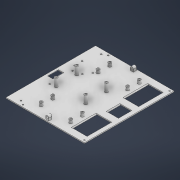
# Autodesk Inventor part: Obenplatte_hinten
Saved by Autodesk Inventor 2021 (Build 250183000, 183)
## iProperties
Created: 2021-02-01
Part Number: Obenplatte_hinten
Material: Generisch
Document SubType Name: Modeling
Designer: laure
Density: 1 g/cm^3
Appearance: Vorgabe
Author: laure
## iProperties of the stored document _3D-Druck.ipt
Created: 2021-02-04
Part Number: _3D-Druck
Material: Generisch
Document SubType Name: Modeling
Designer: Ctroi
Density: 1 g/cm^3
Appearance: Vorgabe
Author: Ctroi
Autodesk Inventor part; units mm, degrees
ref_plane "YZ Plane" through (0, 0, 0) normal (1, 0, 0) x (0, 1, 0)
ref_plane "XZ Plane" through (0, 0, 0) normal (0, 1, 0) x (-1, 0, 0)
ref_plane "XY Plane" through (0, 0, 0) normal (0, 0, 1) x (1, 0, 0)
sketch "Skizze1" plane through (0, 0, 0) normal (0, 1, 0) x (-1, 0, 0)
  line L0 (87.5, -100) -> (-87.5, -100)
  line L1 (-87.5, -100) -> (-87.5, 100)
  line L2 (-87.5, 100) -> (87.5, 100)
  line L3 (87.5, 100) -> (87.5, -100)
  line L4 (0, -140) -> (0, 140) projected
  line L5 (-122.5, 0) -> (122.5, 0) projected
  point P0 (0, 0)
  dimension "d0" = 175
  dimension "d1" = 200
  constraints: 8 end point, 2 parallel, 1 horizontal, 1 perpendicular, 2 other
  measures "d0" distance of L1.end L2.end
  measures "d1" distance of L0.end L1.end
extrude "Extrusion1" add sketch "Skizze1" along normal blind 2
sketch "Skizze2" plane through (0, 2, 0) normal (0, 1, 0) x (1, 0, 0)
  circle A0 centre (-54.5, 95) radius 1.6
  line L0 (0, 140) -> (0, -140) projected
  line L1 (122.5, 0) -> (-122.5, 0) projected
  line L2 (87.5, 100) -> (-87.5, 100) projected
  circle A1 centre (82.5, 95) radius 1.6
  circle A2 centre (-54.5, -95) radius 1.6
  circle A3 centre (82.5, -95) radius 1.6
  line L3 (-87.5, 100) -> (-87.5, -100) projected
  line L4 (87.5, -100) -> (87.5, 100) projected
  point P0 (0, 0)
  dimension "d4" = 3.2
  dimension "d6" = 5
  dimension "d7" = 3.2
  dimension "d9" = 5
  dimension "d40" = 33
  dimension "d41" = 5
  constraints: 4 centre point, 2 symmetric about line, 2 other
  measures "d4" diameter of A0
  measures "d6" distance from line of A0.centre L2
  measures "d7" diameter of A1
  measures "d9" distance from line of L2 A1.centre
  measures "d40" distance from line of L3 A0.centre
  measures "d41" distance from line of L4 A1.centre
extrude "Extrusion2" cut sketch "Skizze2" against normal up to surface (2 mm away) contours A0 | A1 | A2 | A3
sketch "Skizze3" plane through (0, 2, 0) normal (0, 1, 0) x (1, 0, 0)
  line L0 (87.5, -100) -> (87.5, 100) projected
  line L1 (-87.5, -100) -> (87.5, -100) projected
  line L2 (87.5, 100) -> (-87.5, 100) projected
  circle A0 centre (-64.5, 89.5) radius 1.6
  line L3 (-87.5, 100) -> (-87.5, -100) projected
  circle A1 centre (-64.5, 25.5) radius 1.6
  circle A2 centre (-64.5, -25.5) radius 1.6
  circle A3 centre (-64.5, -89.5) radius 1.6
  point P0 (0, 0)
  dimension "d26" = 3.2
  dimension "d27" = 23
  dimension "d28" = 10.5
  dimension "d29" = 3.2
  dimension "d30" = 23
  dimension "d31" = 74.5
  dimension "d32" = 3.2
  dimension "d33" = 23
  dimension "d34" = 74.5
  dimension "d35" = 3.2
  dimension "d36" = 10.5
  dimension "d37" = 23
  constraints: 4 centre point
  measures "d26" diameter of A0
  measures "d27" distance from line of L3 A0.centre
  measures "d28" distance from line of L2 A0.centre
  measures "d29" diameter of A1
  measures "d30" distance from line of L3 A1.centre
  measures "d31" distance from line of L2 A1.centre
  measures "d32" diameter of A2
  measures "d33" distance from line of L3 A2.centre
  measures "d34" distance from line of L1 A2.centre
  measures "d35" diameter of A3
  measures "d36" distance from line of L1 A3.centre
  measures "d37" distance from line of L3 A3.centre
extrude "Extrusion4" cut sketch "Skizze3" against normal up to surface (2 mm away) contours A0 | A1 | A2 | A3
sketch "Skizze4" plane through (0, 2, 0) normal (0, 1, 0) x (1, 0, 0)
  line L0 (-82.5, -12) -> (-72.5, -12)
  line L1 (-72.5, -12) -> (-72.5, 12)
  line L2 (-72.5, 12) -> (-82.5, 12)
  line L3 (-82.5, 12) -> (-82.5, -12)
  line L4 (-82.5, -12) -> (-72.5, 12) construction
  line L5 (-72.5, -12) -> (-82.5, 12) construction
  line L6 (-87.5, 100) -> (-87.5, -100) projected
  line L7 (87.5, 100) -> (-87.5, 100) projected
  point P0 (0, 0)
  point P1 (-77.5, 0)
  dimension "d42" = 10
  dimension "d43" = 24
  dimension "d44" = 5
  dimension "d45" = 88
  constraints: 12 end point, 2 midpoint, 2 parallel, 1 horizontal, 1 perpendicular
  measures "d42" distance of L2.end L1.end
  measures "d43" distance of L1.end L0.end
  measures "d44" distance between parallel lines of L6 L3
  measures "d45" distance between parallel lines of L7 L2
extrude "Extrusion5" cut sketch "Skizze4" against normal up to surface (2 mm away)
fillet "Rundung1" radius 2 1 edges at (-82.5, 0, 0)
fillet "Rundung2" radius 2 1 edges at (-72.5, 2, 0)
sketch "Skizze5" plane through (0, 2, 0) normal (0, 1, 0) x (1, 0, 0)
  circle A0 centre (-32.5, 76.5) radius 3.5
  circle A1 centre (33.5, 76.5) radius 3.5
  circle A2 centre (-32.5, 50.5) radius 3.5
  circle A3 centre (33.5, 50.5) radius 3.5
  line L0 (87.5, 100) -> (-87.5, 100) projected
  line L1 (-87.5, 100) -> (-87.5, -100) projected
  line L2 (45.5, 85) -> (78.5, 85)
  line L3 (78.5, 85) -> (78.5, 30)
  line L4 (78.5, 30) -> (45.5, 30)
  line L5 (45.5, 30) -> (45.5, 85)
  line L6 (122.5, 0) -> (-122.5, 0) projected
  circle A4 centre (-32.5, -76.5) radius 3.5
  circle A5 centre (33.5, -76.5) radius 3.5
  circle A6 centre (-32.5, -50.5) radius 3.5
  circle A7 centre (33.5, -50.5) radius 3.5
  line L7 (45.5, -85) -> (78.5, -85)
  line L8 (78.5, -85) -> (78.5, -30)
  line L9 (78.5, -30) -> (45.5, -30)
  line L10 (45.5, -30) -> (45.5, -85)
  circle A8 centre (-52.5, 23) radius 3.5
  circle A9 centre (-52.5, -23) radius 3.5
  circle A10 centre (13.5, 23) radius 3.5
  circle A11 centre (13.5, -23) radius 3.5
  line L11 (53.5, 15) -> (78.5, 15)
  line L12 (78.5, 15) -> (78.5, -15)
  line L13 (78.5, -15) -> (53.5, -15)
  line L14 (53.5, -15) -> (53.5, 15)
  line L15 (87.5, -100) -> (87.5, 100) projected
  point P0 (0, 0)
  dimension "d50" = 7
  dimension "d51" = 7
  dimension "d52" = 7
  dimension "d53" = 7
  dimension "d54" = 23.5
  dimension "d55" = 23.5
  dimension "d56" = 55
  dimension "d57" = 66
  dimension "d58" = 55
  dimension "d59" = 66
  dimension "d60" = 26
  dimension "d61" = 26
  dimension "d62" = 33
  dimension "d63" = 12
  dimension "d64" = 15
  dimension "d65" = 55
  dimension "d81" = 7
  dimension "d82" = 7
  dimension "d83" = 7
  dimension "d84" = 7
  dimension "d85" = 35
  dimension "d86" = 35
  dimension "d87" = 46
  dimension "d88" = 46
  dimension "d89" = 23
  dimension "d90" = 23
  dimension "d91" = 66
  dimension "d92" = 66
  dimension "d93" = 25
  dimension "d94" = 30
  dimension "d95" = 9
  constraints: 24 end point, 12 centre point, 8 symmetric about line, 4 parallel, 2 horizontal, 2 perpendicular, 5 other
  measures "d50" diameter of A0
  measures "d51" diameter of A1
  measures "d52" diameter of A2
  measures "d53" diameter of A3
  measures "d54" distance from line of L0 A0.centre
  measures "d55" distance from line of L0 A1.centre
  measures "d56" distance from line of L1 A0.centre
  measures "d57" distance of A0.centre A1.centre
  measures "d58" distance from line of L1 A2.centre
  measures "d59" distance of A2.centre A3.centre
  measures "d60" distance of A0.centre A2.centre
  measures "d61" distance of A1.centre A3.centre
  measures "d62" distance of L3.end L4.end
  measures "d63" distance from line of A1.centre L5
  measures "d64" distance between parallel lines of L0 L2
  measures "d65" distance between parallel lines of L2 L4
  measures "d81" diameter of A8
  measures "d82" diameter of A9
  measures "d83" diameter of A10
  measures "d84" diameter of A11
  measures "d85" distance from line of L1 A9.centre
  measures "d86" distance from line of L1 A8.centre
  measures "d87" distance of A8.centre A9.centre
  measures "d88" distance of A10.centre A11.centre
  measures "d89" distance from line of L6 A10.centre
  measures "d90" distance from line of L6 A8.centre
  measures "d91" distance of A10.centre A8.centre
  measures "d92" distance of A9.centre A11.centre
  measures "d93" distance of L12.end L13.end
  measures "d94" distance of L11.end L12.end
  measures "d95" distance between parallel lines of L15 L12
extrude "Extrusion6" add sketch "Skizze5" along normal blind 7 contours A0 | A1 | A2 | A3 | A4 | A5 | A6 | A7
extrude "Extrusion8" cut sketch "Skizze5" against normal up to surface (2 mm away) contours L12 L13 L14 L6 | L6 L14 L11 L12 | L2 L3 L4 L5 | L10 L9 L8 L7
fillet "Rundung3" radius 2 3 edges at (45.5, 2, -57.5) (45.5, 2, 57.5) (53.5, 2, 0)
extrude "Extrusion9" add sketch "Skizze5" along normal blind 18 contours A8 | A9 | A10 | A11
sketch "Skizze6" plane through (-32.5, 9, -76.5) normal (0, 1, 0) x (1, 0, 0)
  circle A0 centre (0, 0) radius 3.5 projected
  circle A1 centre (0, -26) radius 3.5 projected
  circle A2 centre (66, -26) radius 3.5 projected
  circle A3 centre (66, 0) radius 3.5 projected
  circle A4 centre (66, -127) radius 3.5 projected
  circle A5 centre (66, -153) radius 3.5 projected
  circle A6 centre (0, -153) radius 3.5 projected
  circle A7 centre (0, -127) radius 3.5 projected
  circle A8 centre (0, 0) radius 2
  circle A9 centre (0, -26) radius 2
  circle A10 centre (66, -26) radius 2
  circle A11 centre (66, 0) radius 2
  circle A12 centre (0, -127) radius 3.5 projected
  circle A13 centre (0, -127) radius 2
  circle A14 centre (0, -153) radius 2
  circle A15 centre (66, -127) radius 3.5 projected
  circle A16 centre (66, -127) radius 2
  circle A17 centre (66, -153) radius 2
  point P0 (32.5, -76.5)
  dimension "d68" = 4
  dimension "d69" = 4
  dimension "d70" = 4
  dimension "d71" = 4
  dimension "d72" = 4
  dimension "d73" = 4
  dimension "d74" = 4
  dimension "d75" = 4
  constraints: 8 centre point, 8 coincident
  measures "d68" diameter of A8
  measures "d69" diameter of A9
  measures "d70" diameter of A10
  measures "d71" diameter of A11
  measures "d72" diameter of A13
  measures "d73" diameter of A14
  measures "d74" diameter of A16
  measures "d75" diameter of A17
extrude "Extrusion7" cut sketch "Skizze6" against normal blind 5 contours A8 | A9 | A10 | A11 | A13 | A14 | A16 | A17
sketch "Skizze8" plane through (-52.5, 20, -23) normal (0, 1, 0) x (1, 0, 0)
  circle A0 centre (0, 0) radius 3.5 projected
  circle A1 centre (66, 0) radius 3.5 projected
  circle A2 centre (66, -46) radius 3.5 projected
  circle A3 centre (0, -46) radius 3.5 projected
  circle A4 centre (0, 0) radius 3.5 projected
  circle A5 centre (0, 0) radius 2
  circle A6 centre (66, 0) radius 3.5 projected
  circle A7 centre (66, 0) radius 2
  circle A8 centre (66, -46) radius 3.5 projected
  circle A9 centre (66, -46) radius 2
  circle A10 centre (0, -46) radius 3.5 projected
  circle A11 centre (0, -46) radius 2
  point P0 (52.5, -23)
  dimension "d98" = 4
  dimension "d99" = 4
  dimension "d100" = 4
  dimension "d101" = 4
  constraints: 4 centre point, 4 coincident
  measures "d98" diameter of A5
  measures "d99" diameter of A7
  measures "d100" diameter of A9
  measures "d101" diameter of A11
extrude "Extrusion10" cut sketch "Skizze8" against normal blind 5 contours A5 | A7 | A9 | A11
sketch "Skizze9" plane through (0, 2, 0) normal (0, 1, 0) x (1, 0, 0)
  circle A0 centre (-52.5, 22.75) radius 1.75
  circle A1 centre (-32.5, 51.5) radius 1
  line L0 (-52.5, 22.75) -> (-32.5, 51.5)
  circle A2 centre (-47.354, 30.1473) radius 1.6
  circle A3 centre (-37.646, 44.1027) radius 1.6
  circle A4 centre (-42.5, 37.125) radius 0.1
  circle A5 centre (-72.5, 55) radius 1.6
  circle A6 centre (-72.5, 38) radius 1.6
  line L1 (-87.5, 100) -> (-87.5, -100) projected
  line L2 (122.5, 0) -> (-122.5, 0) projected
  line L3 (87.5, 100) -> (-87.5, 100) projected
  circle A7 centre (-32.5, 50.5) radius 3.5 projected
  circle A8 centre (-52.5, 23) radius 3.5 projected
  point P0 (0, 0)
  dimension "d104" = 3.2
  dimension "d105" = 3.2
  dimension "d106" = 13.8
  dimension "d107" = 0.2
  dimension "d108" = 6.8
  dimension "d109" = 3.2
  dimension "d110" = 3.2
  dimension "d111" = 15
  dimension "d112" = 15
  dimension "d113" = 17
  dimension "d134" = 55.8973
  dimension "d135" = 49.8541
  dimension "d136" = 40.1459
  dimension "d137" = 45
  dimension "d138" = 1.5
  dimension "d139" = 1.5
  constraints: 7 centre point, 2 end point, 2 point on line, 1 coincident, 1 midpoint
  measures "d104" diameter of A2
  measures "d105" diameter of A3
  measures "d107" diameter of A4
  measures "d109" diameter of A5
  measures "d110" diameter of A6
  measures "d111" distance from line of L1 A6.centre
  measures "d112" distance from line of L1 A5.centre
  measures "d113" distance of A5.centre A6.centre
  measures "d134" distance from line of L3 A3.centre
  measures "d135" distance from line of L1 A3.centre
  measures "d136" distance from line of L1 A2.centre
  measures "d137" distance from line of L3 A5.centre
extrude "Extrusion11" cut sketch "Skizze9" against normal up to surface (2 mm away) contours A2 L0 | L0 A2 | A3 L0 | L0 A3 | A5 | A6
sketch "Skizze10" plane through (0, 2, 0) normal (0, 1, 0) x (1, 0, 0)
  line L0 (-1, -90.8) -> (6, -90.8)
  line L1 (6, -90.8) -> (6, -97.8)
  line L2 (6, -97.8) -> (-1, -97.8)
  line L3 (-1, -97.8) -> (-1, -90.8)
  line L4 (-87.5, -100) -> (87.5, -100) projected
  line L5 (87.5, -100) -> (87.5, 100) projected
  line L6 (122.5, 0) -> (-122.5, 0) projected
  line L7 (-1, 90.8) -> (6, 90.8)
  line L8 (6, 90.8) -> (6, 97.8)
  line L9 (6, 97.8) -> (-1, 97.8)
  line L10 (-1, 97.8) -> (-1, 90.8)
  point P0 (0, 0)
  dimension "d117" = 7
  dimension "d118" = 7
  dimension "d119" = 2.2
  dimension "d120" = 81.5
  constraints: 16 end point, 4 symmetric about line, 2 parallel, 1 horizontal, 1 perpendicular
  measures "d117" distance of L1.end L2.end
  measures "d118" distance of L0.end L1.end
  measures "d119" distance between parallel lines of L4 L2
  measures "d120" distance between parallel lines of L5 L1
extrude "Extrusion12" add sketch "Skizze10" along normal blind 9
sketch "Skizze11" plane through (-1, 2, 97.8) normal (0, 0, 1) x (1, 0, 0)
  circle A0 centre (3.5, 5) radius 2
  line L0 (7, 0) -> (0, 0) projected
  line L1 (7, 0) -> (7, 9) projected
  point P0 (1, -2)
  dimension "d123" = 4
  dimension "d124" = 5
  dimension "d125" = 3.5
  constraints: 1 centre point
  measures "d123" diameter of A0
  measures "d124" distance from line of L0 A0.centre
  measures "d125" distance from line of L1 A0.centre
extrude "Extrusion13" cut sketch "Skizze11" against normal blind 5
sketch "Skizze12" plane through (6, 2, -97.8) normal (0, 0, -1) x (-1, 0, 0)
  circle A0 centre (3.5, 5) radius 2
  line L0 (7, 0) -> (0, 0) projected
  line L1 (7, 0) -> (7, 9) projected
  point P0 (6, -2)
  dimension "d128" = 4
  dimension "d129" = 5
  dimension "d130" = 3.5
  constraints: 1 centre point
  measures "d128" diameter of A0
  measures "d129" distance from line of L0 A0.centre
  measures "d130" distance from line of L1 A0.centre
extrude "Extrusion14" cut sketch "Skizze12" against normal blind 5
fillet "Rundung4" radius 3.5 4 edges at (6, 11, -94.3) (-1, 11, -94.3) (-1, 11, 94.3) (6, 11, 94.3)
